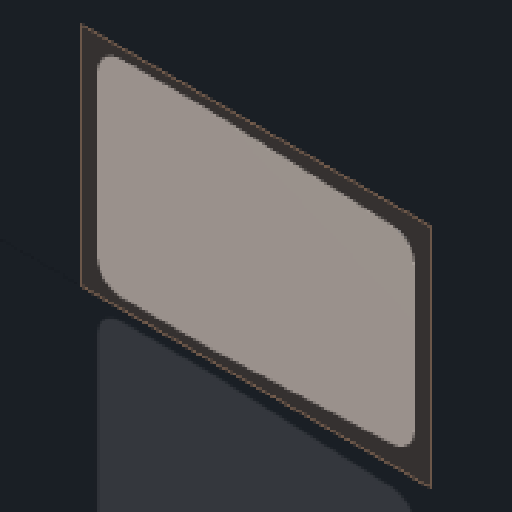
# Autodesk Inventor part: CARCASA_ALUM_4
Saved by Autodesk Inventor 2024.3 (Build 283343000, 343)
## iProperties
Created: 2024-05-15
Part Number: CARCASA_ALUM_4
Material: Generic
Document SubType Name: Sheet Metal
Designer: Niler
Density: 1 g/cm^3
Sheet Metal Rule: Default_mm
Appearance: Default
Author: Niler
Autodesk Inventor part; units mm, degrees
ref_plane "YZ Plane" through (0, 0, 0) normal (1, 0, 0) x (0, 1, 0)
ref_plane "XZ Plane" through (0, 0, 0) normal (0, 1, 0) x (-1, 0, 0)
ref_plane "XY Plane" through (0, 0, 0) normal (0, 0, 1) x (1, 0, 0)
ref_plane "Work Plane1" through (0, 0, 0) normal (0, 0, 1) x (1, 0, 0)
sketch "Sketch1" plane through (0, 0, 0) normal (0, 0, 1) x (1, 0, 0)
  arc A0 (-0.0454, -1100) -> (0.0454, -1099.9979) centre (-0.0454, -1098) ccw
  line L0 (0.0454, -1099.9979) -> (975.903, -1055.6408)
  arc A1 (975.903, -1055.6408) -> (1100, -925.7749) centre (970, -925.7749) ccw
  line L1 (1100, -174.2251) -> (1100, -925.7749)
  arc A2 (1100, -174.2251) -> (975.903, -44.3592) centre (970, -174.2251) ccw
  line L2 (0.0454, -0.0021) -> (975.903, -44.3592)
  arc A3 (0.0454, -0.0021) -> (-0.0454, 0) centre (-0.0454, -2) ccw
  line L3 (-0.0454, 0) -> (-470, 0)
  arc A4 (-470, 0) -> (-600, -130) centre (-470, -130) ccw
  line L4 (-600, -970) -> (-600, -130)
  arc A5 (-600, -970) -> (-470, -1100) centre (-470, -970) ccw
  line L5 (-0.0454, -1100) -> (-470, -1100)
  point P0 (0, 0)
extrude "Plate1" add sketch "Sketch1" against normal blind 1.5
equation "\"d0\" = Thickness"
equation "\"BendRadius\" = Thickness"
equation "\"BendReliefWidth\" = Thickness"
equation "\"BendReliefDepth\" = 0.5 * Thickness"
equation "\"CornerReliefSize\" = 4 * Thickness"
equation "\"MinimumRemnant\" = 2 * Thickness"
equation "\"TransitionRadius\" = BendRadius"
equation "\"JacobiRadiusSize\" = BendRadius"
equation "\"GapSize\" = Thickness"
equation "\"Thickness\" = 1.5"
body "Solid1"
